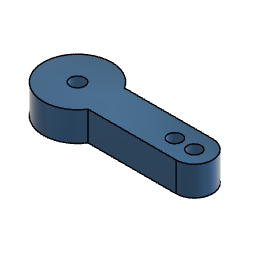
Servo_Horn v1 (Autodesk Fusion 360 design; units mm, degrees)
Autodesk Fusion 360 part; units mm, degrees
sketch "Skizze1" plane through (0, 0, 0) normal (0, 1, 0) x (1, 0, 0)
  circle A0 centre (0, 0) radius 1.5
  circle A1 centre (20, 0) radius 1.4
  circle A2 centre (24, 0) radius 1.4
  line L0 (0, 0) -> (24, 0) construction
  line L1 (24, 3.75) -> (5.9108, 3.75)
  line L2 (24, -3.75) -> (5.9108, -3.75)
  arc A3 (24, -3.75) -> (24, 3.75) centre (24, 0) ccw
  arc A4 (5.9108, 3.75) -> (5.9108, -3.75) centre (0, 0) ccw
  dimension "d1" = 3
  dimension "d2" = 2.8
  dimension "d3" = 2.8
  dimension "d4" = 20
  dimension "d5" = 4
  dimension "d6" = 14
  dimension "d7" = 7.5
  constraint coincident A0.centre L0.start
  constraint coincident A2.centre L0.end
  constraint horizontal L0
  constraint coincident A1.centre L0
  constraint concentric A0 A4
  constraint concentric A2 A3
  constraint tangent L1 A3
  constraint horizontal L1
  constraint tangent L2 A3
  constraint horizontal L2
  measures "d1" diameter of A0
  measures "d2" diameter of A1
  measures "d3" diameter of A2
  measures "d4" distance of A0.centre A1.centre
  measures "d5" distance of A1.centre A2.centre
  measures "d6" diameter of A4
  measures "d7" diameter of A3
extrude "Extrusion1" add sketch "Skizze1" along normal blind 6
